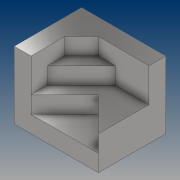
# Autodesk Inventor part: 19
Saved by Autodesk Inventor 2020.2 (Build 242310000, 310)
## iProperties
Created: 2020-09-17
Part Number: 19
Material: 鋼、碳鋼
Document SubType Name: Modeling
Designer: user
Density: 7.85 g/cm^3
Appearance: 半拋光
Mass: 427.825 g
Surface Area: 111.899 cm^2
Volume: 54.5 cm^3
Author: user
Autodesk Inventor part; units mm, degrees
ref_plane "YZ Plane" through (0, 0, 0) normal (1, 0, 0) x (0, 1, 0)
ref_plane "XZ Plane" through (0, 0, 0) normal (0, 1, 0) x (-1, 0, 0)
ref_plane "XY Plane" through (0, 0, 0) normal (0, 0, 1) x (1, 0, 0)
sketch "草圖1" plane through (0, 0, 0) normal (0, 1, 0) x (-1, 0, 0)
  line L0 (0, 0) -> (-50, 0)
  line L1 (-50, 0) -> (-50, 40)
  line L2 (-50, 40) -> (0, 40)
  line L3 (0, 40) -> (0, 0)
  dimension "d0" = 50
  dimension "d1" = 40
  constraints: 8 end point, 2 parallel, 1 horizontal, 1 perpendicular
  measures "d0" distance of L0.start L0.end
  measures "d1" distance of L2.end L0.start
extrude "擠出1" add sketch "草圖1" along normal blind 40
sketch "草圖3" plane through (0, 40, 0) normal (0, 1, 0) x (1, 0, 0)
  line L0 (50, 0) -> (50, -40) projected
  line L1 (50, -40) -> (0, -40) projected
  line L2 (0, -40) -> (0, 0) projected
  line L3 (0, 0) -> (50, 0) projected
  line L4 (10, -40) -> (10, -20)
  line L5 (10, -20) -> (20, -10)
  line L6 (20, -10) -> (50, -10)
  line L7 (50, -40) -> (50, 0) projected
  dimension "d10" = 10
  dimension "d11" = 10
  dimension "d12" = 30
  dimension "d13" = 20
  constraints: 6 end point, 2 perpendicular, 2 point on line
  measures "d10" distance between parallel lines of L4 L2
  measures "d11" distance between parallel lines of L3 L6
  measures "d12" distance of L5.end L6.end
  measures "d13" distance of L4.start L4.end
extrude "擠出3" cut sketch "草圖3" against normal blind 20 contours L0 L1 L4 L5 L6
sketch "草圖4" plane through (0, 20, 0) normal (0, 1, 0) x (1, 0, 0)
  line L0 (50, -10) -> (20, -10) projected
  line L1 (20, -10) -> (10, -20) projected
  line L2 (10, -20) -> (10, -40) projected
  line L3 (50, -40) -> (10, -40) projected
  line L4 (50, -10) -> (50, -40) projected
  line L5 (50, 0) -> (50, -10) projected
  line L6 (0, 0) -> (50, 0) projected
  line L7 (0, -40) -> (0, 0) projected
  line L8 (10, -40) -> (0, -40) projected
  line L9 (50, -40) -> (10, -40) projected
  line L10 (10, -40) -> (30, -20)
  line L11 (30, -20) -> (50, -40)
  dimension "d16" = 20
  dimension "d17" = 20
  constraints: 4 end point
  measures "d16" distance from line of L4 L10.end
  measures "d17" distance from line of L10.end L3
extrude "擠出4" cut sketch "草圖4" against normal blind 10 contours L3 L10 L11
sketch "草圖5" plane through (0, 20, 0) normal (0, 1, 0) x (1, 0, 0)
  line L0 (50, -10) -> (20, -10) projected
  line L1 (20, -10) -> (10, -20) projected
  line L2 (10, -20) -> (10, -40) projected
  line L3 (10, -40) -> (0, -40) projected
  line L4 (0, -40) -> (0, 0) projected
  line L5 (0, 0) -> (50, 0) projected
  line L6 (50, 0) -> (50, -10) projected
  line L7 (50, -10) -> (50, -40) projected
  line L8 (50, -40) -> (30, -20) projected
  line L9 (30, -20) -> (10, -40) projected
  line L10 (10, -40) -> (10, -20) projected
  line L11 (10, -30) -> (30, -10)
  line L12 (20, -10) -> (50, -10) projected
  point P0 (30, -10)
  dimension "d20" = 10
  dimension "d21" = 20
  constraints: 2 end point, 1 midpoint, 1 point on line
  measures "d20" distance from line of L3 L11.start
  measures "d21" distance from line of L6 L11.end
extrude "擠出5" add sketch "草圖5" along normal blind 10 contours L11 L2 L1 L0
